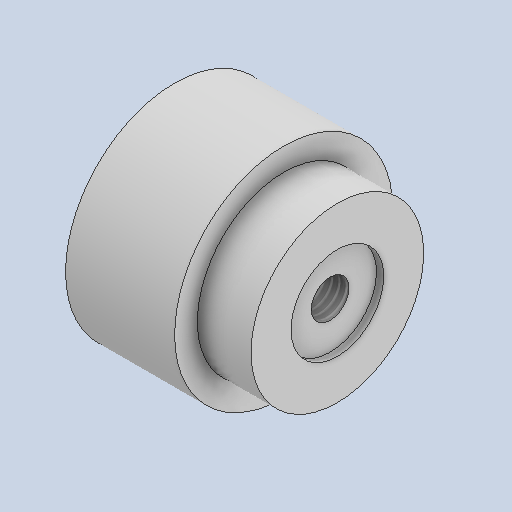
# Autodesk Inventor part: SpringCompensation_Outside_DrivenPart
Saved by Autodesk Inventor 2022 (Build 260153000, 153)
## iProperties
Created: 2022-10-13
Part Number: SpringCompensation_Outside_DrivenPart
Material: Generisch
Document SubType Name: Modeling
Designer: alexw
Density: 1 g/cm^3
Appearance: Vorgabe
Mass: 6.8066 g
Surface Area: 23.826 cm^2
Volume: 6.8066 cm^3
Author: alexw
Autodesk Inventor part; units mm, degrees
ref_plane "YZ Plane" through (0, 0, 0) normal (1, 0, 0) x (0, 1, 0)
ref_plane "XZ Plane" through (0, 0, 0) normal (0, 1, 0) x (-1, 0, 0)
ref_plane "XY Plane" through (0, 0, 0) normal (0, 0, 1) x (1, 0, 0)
sketch "Skizze1" plane through (0, 0, 0) normal (0, 0, 1) x (1, 0, 0)
  line L0 (0, 0) -> (0, 12)
  line L1 (0, 12) -> (12, 12)
  line L2 (12, 12) -> (12, 9.5)
  line L3 (12, 9.5) -> (17.9, 9.5)
  line L4 (17.9, 9.5) -> (17.9, 5)
  line L5 (0, 0) -> (17.1, 0)
  line L6 (17.9, 5) -> (17.1, 5)
  line L7 (17.1, 5) -> (17.1, 0)
  dimension "d0" = 19
  dimension "d1" = 24
  dimension "d2" = 5.9
  dimension "d3" = 12
  dimension "d12" = 10
  dimension "d13" = 5.1
  constraints: 16 end point, 5 perpendicular, 2 horizontal, 1 vertical
  measures "d0" diameter of L3 L5
  measures "d1" diameter of L1 L5
  measures "d2" distance between parallel lines of L4 L2
  measures "d3" distance between parallel lines of L0 L2
  measures "d12" diameter of L6 L5
  measures "d13" distance between parallel lines of L2 L7
revolve "Umdrehung1" add sketch "Skizze1" angle 360 about axis through (0, 0, 0) along (1, 0, 0)
sketch "Skizze2" plane through (0, 0, 0) normal (-1, 0, 0) x (0, 0, 1)
  point P0 (0, 0)
  point P1 (0, 0)
  constraints: 1 coincident
hole "Bohrung1" at (0, 0, 0) direction (1, 0, 0) diameter 4.134 end through all thread size "M5x0.8" class "6H" standard "ISO Metric profile"
feature "Verdickung1" [suppressed]
thicken "Verdickung2" operation add thickness 0.1 both sides no extend neighbours yes toward (0, 0.9870503, -0.1604113) faces at (17.3667, 4.9353, -0.8021)
